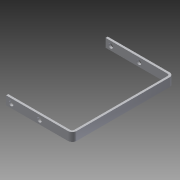
# Autodesk Inventor part: tie-together tier 1
Saved by Autodesk Inventor 2013 (Build 170138000, 138)
## iProperties
Created: 2013-01-24
Part Number: tie-together tier 1
Material: Aluminum 6061
Document SubType Name: Sheet Metal
Designer: Arpan
Density: 2.71 g/cm^3
Sheet Metal Rule: Default
Mass: 35.6654 g
Surface Area: 107.751 cm^2
Volume: 13.1607 cm^3
Flat Pattern Width: 1.27 cm
Flat Pattern Length: 33.6562 cm
Flat Pattern Area: 42.7434 cm^2
Sheet Metal Width: 0.500 in
Sheet Metal Length: 13.250 in
Sheet Metal Area: 6.625 in^2
Author: Arpan
Autodesk Inventor part; units mm, degrees
note: some values were not read from the file. Left out: dimensions or parameters whose unit could not be read.
ref_plane "YZ Plane" through (0, 0, 0) normal (1, 0, 0) x (0, 1, 0)
ref_plane "XZ Plane" through (0, 0, 0) normal (0, 1, 0) x (-1, 0, 0)
ref_plane "XY Plane" through (0, 0, 0) normal (0, 0, 1) x (1, 0, 0)
sketch "Sketch1" plane through (0, 0, 0) normal (0, 0, 1) x (1, 0, 0)
  line L0 (0, 0) -> (336.562362, 0)
  line L1 (336.562362, -12.7) -> (0, -12.7)
  line L2 (0, 0) -> (95.513688, 0)
  line L3 (95.513688, 0) -> (95.513688, -1.5875)
  line L4 (95.513688, -1.5875) -> (94.719938, -1.5875)
  line L5 (94.719938, -1.5875) -> (94.719938, 0)
  line L6 (95.513688, -1.5875) -> (96.307438, -1.5875)
  line L7 (96.307438, -1.5875) -> (96.307438, 0)
  line L8 (95.513688, -12.7) -> (95.513688, -11.1125)
  line L9 (95.513688, -11.1125) -> (94.719938, -11.1125)
  line L10 (94.719938, -11.1125) -> (94.719938, -12.7)
  line L11 (95.513688, -11.1125) -> (96.307438, -11.1125)
  line L12 (96.307438, -11.1125) -> (96.307438, -12.7)
  line L13 (336.562362, 0) -> (241.058362, 0)
  line L14 (241.058362, 0) -> (241.058362, -1.5875)
  line L15 (241.058362, -1.5875) -> (241.852112, -1.5875)
  line L16 (241.852112, -1.5875) -> (241.852112, 0)
  line L17 (241.058362, -1.5875) -> (240.264612, -1.5875)
  line L18 (240.264612, -1.5875) -> (240.264612, 0)
  line L19 (241.058362, -12.7) -> (241.058362, -11.1125)
  line L20 (241.058362, -11.1125) -> (241.852112, -11.1125)
  line L21 (241.852112, -11.1125) -> (241.852112, -12.7)
  line L22 (241.058362, -11.1125) -> (240.264612, -11.1125)
  line L23 (240.264612, -11.1125) -> (240.264612, -12.7)
  dimension "d1" = 91.9226
  constraints: 12 end point, 2 perpendicular, 2 point on line, 1 horizontal, 1 parallel
  measures "d1" distance of L0.start L0.end
sketch "Sketch1 outline for Plate5" plane through (0, 0, 0) normal (0, 0, 1) x (1, 0, 0)
  line L0 (-91.9226, 0) -> (0, 0)
  line L1 (-91.9226, 12.7) -> (-91.9226, 0)
  line L2 (-84.4296, 12.7) -> (-91.9226, 12.7)
  line L3 (-42.418, 12.7) -> (-84.4296, 12.7)
  line L4 (0, 12.7) -> (-42.418, 12.7)
  line L5 (0, 0) -> (0, 12.7)
extrude "Plate5" add sketch "Sketch1 outline for Plate5" along normal blind 3.175
sketch "Sketch6" plane through (3.175, 0, -3.175) normal (1, 0, 0) x (0, 1, 0)
  line L0 (12.7, 0) -> (0, 0)
  line L1 (0, 0) -> (0, -138.3538)
  line L2 (0, -138.3538) -> (12.7, -138.3538)
  line L3 (12.7, -138.3538) -> (12.7, 0)
  constraints: 6 end point, 1 horizontal, 1 perpendicular, 1 vertical
edge flange "Flange4" height 144.7038 angle 90 thickness 3.175 bend radius 3.175 thickness toward (1, 0, 0) relief tear relief width 3.175 relief depth 1.5875 edges at (0, 6.35, 0) wall of the first edge with corners at (3.175, 12.7, -3.175) (3.175, 0, -3.175) (3.175, 0, -141.5288) (3.175, 12.7, -141.5288)
bend "Bend4"
corner "Corner4"
sketch "Sketch7" plane through (0, 0, -144.7038) normal (0, 0, -1) x (-1, 0, 0)
  line L0 (0, 12.7) -> (0, 0)
  line L1 (0, 0) -> (91.9226, 0)
  line L2 (91.9226, 0) -> (91.9226, 12.7)
  line L3 (91.9226, 12.7) -> (0, 12.7)
  constraints: 6 end point, 1 horizontal, 1 perpendicular, 1 vertical
edge flange "Flange5" height 98.2726 angle 90 thickness 3.175 bend radius 3.175 thickness toward (0, 0, -1) relief tear relief width 3.175 relief depth 1.5875 edges at (3.175, 6.35, -141.5288) wall of the first edge with corners at (0, 12.7, -144.7038) (0, 0, -144.7038) (-91.9226, 0, -144.7038) (-91.9226, 12.7, -144.7038)
bend "Bend5"
corner "Corner5"
sketch "Sketch9" plane through (0, 0, 3.175) normal (0, 0, 1) x (1, 0, 0)
  circle A0 centre (-42.4226, 501.2188) radius 3.3 projected
  circle A1 centre (-84.4226, 501.2188) radius 3.3 projected
extrude "Extrusion3" cut sketch "Sketch9" against normal blind 25374.6
sketch "Sketch10" plane through (-91.9226, 0, -144.7038) normal (0, 0, 1) x (1, 0, 0)
  line L0 (45, 276.1188) -> (45, -384.2812)
  circle A0 centre (7.5, 5.9188) radius 3.3
  circle A1 centre (49.5, 5.9188) radius 3.3
  constraints: 2 centre point, 2 end point, 1 vertical, 6 other
extrude "Extrusion4" cut sketch "Sketch10" along normal mid plane 25374.6
sketch "Sketch2" plane through (336.562362, -12.7, 0) normal (0, 0, 1) x (1, 0, 0)
  line L0 (-95.504, 12.7) -> (0, 12.7)
  line L1 (-95.504, 12.7) -> (-95.504, 11.1125)
  line L2 (-241.048674, 11.1125) -> (-241.048674, 12.7)
  line L3 (-336.562362, 12.7) -> (-241.048674, 12.7)
  line L4 (-241.048674, 12.7) -> (-241.842424, 12.7)
  line L5 (-241.842424, 12.7) -> (-241.842424, 11.1125)
  line L6 (-241.842424, 11.1125) -> (-241.048674, 11.1125)
  line L7 (-95.504, 12.7) -> (-94.71025, 12.7)
  line L8 (-95.504, 11.1125) -> (-94.71025, 11.1125)
  line L9 (-94.71025, 11.1125) -> (-94.71025, 12.7)
  dimension "d14" = 0.79375
  dimension "d15" = 0.79375
  constraints: 12 end point, 2 parallel, 2 perpendicular, 2 point on line
  measures "d14" distance of L2.end L4.end
  measures "d15" distance of L0.start L7.end
equation "\"d43\" = BendReliefWidth"
equation "\"d44\" = BendReliefDepth"
equation "\"d45\" = MinimumRemnant"
equation "\"d46\" = BendRadius"
equation "\"d49\" = BendRadius"
equation "\"d50\" = CornerReliefSize"
equation "\"d51\" = GapSize"
equation "\"d52\" = JacobiRadiusSize"
equation "\"d53\" = BendReliefWidth"
equation "\"d54\" = BendReliefDepth"
equation "\"d55\" = MinimumRemnant"
equation "\"d56\" = BendRadius"
equation "\"d59\" = BendRadius"
equation "\"d60\" = CornerReliefSize"
equation "\"d61\" = GapSize"
equation "\"d62\" = JacobiRadiusSize"
equation "\"BendRadius\" = Thickness"
equation "\"BendReliefWidth\" = Thickness"
equation "\"BendReliefDepth\" = 0.5 * Thickness"
equation "\"CornerReliefSize\" = 4 * Thickness"
equation "\"MinimumRemnant\" = 2 * Thickness"
equation "\"TransitionRadius\" = BendRadius"
equation "\"JacobiRadiusSize\" = BendRadius"
equation "\"GapSize\" = Thickness"
equation "\"d8\" = BendRadius"
equation "\"d42\" = BendRadius"
equation "\"Thickness\" = 3.175"
body "Solid2"
